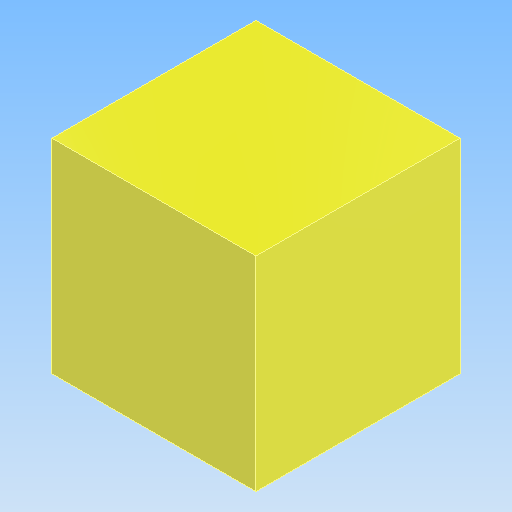
# Autodesk Inventor part: box1
Saved by Autodesk Inventor 2026.1 (Build 301233020, 233B)
## iProperties
RuleStatus: InUse
Created: 2023-10-19
Part Number: box1
Material: Generic
Document SubType Name: Modeling
Designer: e3d
Density: 1 g/cm^3
Appearance: Yellow
Author: e3d
Autodesk Inventor part; units mm, degrees
note: some values were not read from the file. Left out: dimensions or parameters whose unit could not be read.
ref_plane "YZ Plane" through (0, 0, 0) normal (1, 0, 0) x (0, 1, 0)
ref_plane "XZ Plane" through (0, 0, 0) normal (0, 1, 0) x (-1, 0, 0)
ref_plane "XY Plane" through (0, 0, 0) normal (0, 0, 1) x (1, 0, 0)
sketch "Sketch1" plane through (0, 0, 0) normal (0, 0, 1) x (1, 0, 0)
  line L0 (-71.4514, 2.2796) -> (4.7486, 2.2796)
  line L1 (4.7486, 2.2796) -> (4.7486, -73.9204)
  line L2 (4.7486, -73.9204) -> (-71.4514, -73.9204)
  line L3 (-71.4514, -73.9204) -> (-71.4514, 2.2796)
  dimension "d2" = 76.2
  dimension "d3" = 76.2
  constraints: 8 end point, 2 parallel, 1 horizontal, 1 perpendicular
  measures "d2" distance of L0.start L0.end
  measures "d3" distance of L0.end L1.end
extrude "Extrusion1" add sketch "Sketch1" along normal blind 76.2
equation "\"d2\" = Length"
equation "\"d3\" = Height"
equation "\"d0\" = Width"
equation "\"Length\" = 76.2"
equation "\"Width\" = 76.2"
equation "\"Height\" = 76.2"
equation "\"L__\" = Length"
equation "\"W__\" = Width"
equation "\"H__\" = Height"
body "Solid1"
